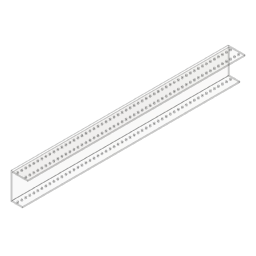
Drivebase Frame v4 (Autodesk Fusion 360 design; units mm, degrees)
Autodesk Fusion 360 part; units mm, degrees
sketch "Sketch1" plane through (0, 0, 0) normal (0, 1, 0) x (1, 0, 0)
  line L0 (-20.3201, -44.3567) -> (29.6862, -44.3567)
  line L1 (13.0174, 33.4308) -> (-20.3201, 33.4308)
  line L2 (-20.3201, 33.4308) -> (-20.3201, -44.3567)
  line L3 (13.0174, 36.6058) -> (-23.4951, 36.6058)
  line L4 (-23.4951, 36.6058) -> (-23.4951, -47.5317)
  line L5 (-23.4951, -47.5317) -> (29.6862, -47.5317)
  line L6 (-23.495, 33.4308) -> (-23.495, 36.6058)
  line L7 (13.0174, 36.6058) -> (13.0174, 33.4308)
  line L8 (29.6862, -47.5317) -> (29.6862, -44.3567)
  dimension "d4" = 53.1812
  dimension "d5" = 84.1375
  dimension "d6" = 36.5125
  constraint horizontal L0
  constraint horizontal L1
  constraint vertical L2
  constraint coincident L1 L6.start
  constraint coincident L3 L6.end
  constraint perpendicular L3 L6
  constraint perpendicular L1 L7
  measures "d4" distance of L4.end L5.end
  measures "d5" distance of L3.end L4.end
  measures "d6" distance of L3.start L3.end
extrude "Extrude1" add sketch "Sketch1" along normal blind 687.3875
sketch "Sketch2" plane through (0, 0, 47.5317) normal (0, 0, 1) x (-1, 0, 0)
  line L0 (23.4951, 0) -> (-29.6862, 0)
  line L1 (-29.6862, 0) -> (-29.6862, -687.3875)
  line L2 (-29.6862, -687.3875) -> (23.4951, -687.3875)
  line L3 (23.4951, -687.3875) -> (23.4951, 0)
  circle A0 centre (-16.9862, -6.35) radius 2.3813
  circle A1 centre (8.4138, -6.35) radius 2.3813
  circle A2 centre (-16.9862, -19.05) radius 2.3813
  circle A3 centre (8.4138, -19.05) radius 2.3813
  circle A4 centre (-16.9862, -31.75) radius 2.3813
  circle A5 centre (8.4138, -31.75) radius 2.3813
  circle A6 centre (-16.9862, -44.45) radius 2.3813
  circle A7 centre (8.4138, -44.45) radius 2.3813
  circle A8 centre (-16.9862, -57.15) radius 2.3813
  circle A9 centre (8.4138, -57.15) radius 2.3813
  circle A10 centre (-16.9862, -69.85) radius 2.3813
  circle A11 centre (8.4138, -69.85) radius 2.3813
  circle A12 centre (-16.9862, -82.55) radius 2.3813
  circle A13 centre (8.4138, -82.55) radius 2.3813
  circle A14 centre (-16.9862, -95.25) radius 2.3813
  circle A15 centre (8.4138, -95.25) radius 2.3813
  circle A16 centre (-16.9862, -107.95) radius 2.3813
  circle A17 centre (8.4138, -107.95) radius 2.3813
  circle A18 centre (-16.9862, -120.65) radius 2.3813
  circle A19 centre (8.4138, -120.65) radius 2.3813
  circle A20 centre (-16.9862, -133.35) radius 2.3813
  circle A21 centre (8.4138, -133.35) radius 2.3813
  circle A22 centre (-16.9862, -146.05) radius 2.3813
  circle A23 centre (8.4138, -146.05) radius 2.3813
  circle A24 centre (-16.9862, -158.75) radius 2.3813
  circle A25 centre (8.4138, -158.75) radius 2.3813
  circle A26 centre (-16.9862, -171.45) radius 2.3813
  circle A27 centre (8.4138, -171.45) radius 2.3813
  circle A28 centre (-16.9862, -184.15) radius 2.3813
  circle A29 centre (8.4138, -184.15) radius 2.3813
  circle A30 centre (-16.9862, -196.85) radius 2.3813
  circle A31 centre (8.4138, -196.85) radius 2.3813
  circle A32 centre (-16.9862, -209.55) radius 2.3813
  circle A33 centre (8.4138, -209.55) radius 2.3813
  circle A34 centre (-16.9862, -222.25) radius 2.3813
  circle A35 centre (8.4138, -222.25) radius 2.3813
  circle A36 centre (-16.9862, -234.95) radius 2.3813
  circle A37 centre (8.4138, -234.95) radius 2.3813
  circle A38 centre (-16.9862, -247.65) radius 2.3813
  circle A39 centre (8.4138, -247.65) radius 2.3813
  circle A40 centre (-16.9862, -260.35) radius 2.3813
  circle A41 centre (8.4138, -260.35) radius 2.3813
  circle A42 centre (-16.9862, -273.05) radius 2.3813
  circle A43 centre (8.4138, -273.05) radius 2.3813
  circle A44 centre (-16.9862, -285.75) radius 2.3813
  circle A45 centre (8.4138, -285.75) radius 2.3813
  circle A46 centre (-16.9862, -298.45) radius 2.3813
  circle A47 centre (8.4138, -298.45) radius 2.3813
  circle A48 centre (-16.9862, -311.15) radius 2.3813
  circle A49 centre (8.4138, -311.15) radius 2.3813
  circle A50 centre (-16.9862, -323.85) radius 2.3813
  circle A51 centre (8.4138, -323.85) radius 2.3813
  circle A52 centre (-16.9862, -336.55) radius 2.3813
  circle A53 centre (8.4138, -336.55) radius 2.3813
  circle A54 centre (-16.9862, -349.25) radius 2.3813
  circle A55 centre (8.4138, -349.25) radius 2.3813
  circle A56 centre (-16.9862, -361.95) radius 2.3813
  circle A57 centre (8.4138, -361.95) radius 2.3813
  circle A58 centre (-16.9862, -374.65) radius 2.3813
  circle A59 centre (8.4138, -374.65) radius 2.3813
  circle A60 centre (-16.9862, -387.35) radius 2.3813
  circle A61 centre (8.4138, -387.35) radius 2.3813
  circle A62 centre (-16.9862, -400.05) radius 2.3813
  circle A63 centre (8.4138, -400.05) radius 2.3813
  circle A64 centre (-16.9862, -412.75) radius 2.3813
  circle A65 centre (8.4138, -412.75) radius 2.3813
  circle A66 centre (-16.9862, -425.45) radius 2.3813
  circle A67 centre (8.4138, -425.45) radius 2.3813
  circle A68 centre (-16.9862, -438.15) radius 2.3813
  circle A69 centre (8.4138, -438.15) radius 2.3813
  circle A70 centre (-16.9862, -450.85) radius 2.3813
  circle A71 centre (8.4138, -450.85) radius 2.3813
  circle A72 centre (-16.9862, -463.55) radius 2.3813
  circle A73 centre (8.4138, -463.55) radius 2.3813
  circle A74 centre (-16.9862, -476.25) radius 2.3813
  circle A75 centre (8.4138, -476.25) radius 2.3813
  circle A76 centre (-16.9862, -488.95) radius 2.3813
  circle A77 centre (8.4138, -488.95) radius 2.3813
  circle A78 centre (-16.9862, -501.65) radius 2.3813
  circle A79 centre (8.4138, -501.65) radius 2.3813
  circle A80 centre (-16.9862, -514.35) radius 2.3813
  circle A81 centre (8.4138, -514.35) radius 2.3813
  circle A82 centre (-16.9862, -527.05) radius 2.3813
  circle A83 centre (8.4138, -527.05) radius 2.3813
  circle A84 centre (-16.9862, -539.75) radius 2.3813
  circle A85 centre (8.4138, -539.75) radius 2.3813
  circle A86 centre (-16.9862, -552.45) radius 2.3813
  circle A87 centre (8.4138, -552.45) radius 2.3813
  circle A88 centre (-16.9862, -565.15) radius 2.3813
  circle A89 centre (8.4138, -565.15) radius 2.3813
  circle A90 centre (-16.9862, -577.85) radius 2.3813
  circle A91 centre (8.4138, -577.85) radius 2.3813
  circle A92 centre (-16.9862, -590.55) radius 2.3813
  circle A93 centre (8.4138, -590.55) radius 2.3813
  circle A94 centre (-16.9862, -603.25) radius 2.3813
  circle A95 centre (8.4138, -603.25) radius 2.3813
  circle A96 centre (-16.9862, -615.95) radius 2.3813
  circle A97 centre (8.4138, -615.95) radius 2.3813
  circle A98 centre (-16.9862, -628.65) radius 2.3813
  circle A99 centre (8.4138, -628.65) radius 2.3813
  circle A100 centre (-16.9862, -641.35) radius 2.3813
  circle A101 centre (8.4138, -641.35) radius 2.3813
  circle A102 centre (-16.9862, -654.05) radius 2.3813
  circle A103 centre (8.4138, -654.05) radius 2.3813
  circle A104 centre (-16.9862, -666.75) radius 2.3813
  circle A105 centre (8.4138, -666.75) radius 2.3813
  circle A106 centre (-16.9862, -679.45) radius 2.3813
  circle A107 centre (8.4138, -679.45) radius 2.3813
  dimension "d9" = 4.7625
  dimension "d12" = 25.4
  dimension "d13" = -12.7
  measures "d9" diameter of A0
hole "Hole1" at (16.9862, 6.35, 47.5317) direction (0, 0, -1) diameter 4.7752 depth 4.7752 tip angle 118
pattern_linear "R-Pattern1" count 54 spacing 12.7 along (0, 1, 0) count 2 spacing 25.4 along (-1, 0, 0) of "Hole1"
sketch "Sketch3" plane through (0, 0, -36.6058) normal (0, 0, -1) x (1, 0, 0)
  line L0 (13.0174, 0) -> (-23.4951, 0)
  line L1 (-23.4951, 0) -> (-23.4951, -687.3875)
  line L2 (-23.4951, -687.3875) -> (13.0174, -687.3875)
  line L3 (13.0174, -687.3875) -> (13.0174, 0)
  circle A0 centre (-8.4075, -6.35) radius 2.3813
  circle A1 centre (-8.4075, -19.05) radius 2.3813
  circle A2 centre (-8.4075, -31.75) radius 2.3813
  circle A3 centre (-8.4075, -44.45) radius 2.3813
  circle A4 centre (-8.4075, -57.15) radius 2.3813
  circle A5 centre (-8.4075, -69.85) radius 2.3813
  circle A6 centre (-8.4075, -82.55) radius 2.3813
  circle A7 centre (-8.4075, -95.25) radius 2.3813
  circle A8 centre (-8.4075, -107.95) radius 2.3813
  circle A9 centre (-8.4075, -120.65) radius 2.3813
  circle A10 centre (-8.4075, -133.35) radius 2.3813
  circle A11 centre (-8.4075, -146.05) radius 2.3813
  circle A12 centre (-8.4075, -158.75) radius 2.3813
  circle A13 centre (-8.4075, -171.45) radius 2.3813
  circle A14 centre (-8.4075, -184.15) radius 2.3813
  circle A15 centre (-8.4075, -196.85) radius 2.3813
  circle A16 centre (-8.4075, -209.55) radius 2.3813
  circle A17 centre (-8.4075, -222.25) radius 2.3813
  circle A18 centre (-8.4075, -234.95) radius 2.3813
  circle A19 centre (-8.4075, -247.65) radius 2.3813
  circle A20 centre (-8.4075, -260.35) radius 2.3813
  circle A21 centre (-8.4075, -273.05) radius 2.3813
  circle A22 centre (-8.4075, -285.75) radius 2.3813
  circle A23 centre (-8.4075, -298.45) radius 2.3813
  circle A24 centre (-8.4075, -311.15) radius 2.3813
  circle A25 centre (-8.4075, -323.85) radius 2.3813
  circle A26 centre (-8.4075, -336.55) radius 2.3813
  circle A27 centre (-8.4075, -349.25) radius 2.3813
  circle A28 centre (-8.4075, -361.95) radius 2.3813
  circle A29 centre (-8.4075, -374.65) radius 2.3813
  circle A30 centre (-8.4075, -387.35) radius 2.3813
  circle A31 centre (-8.4075, -400.05) radius 2.3813
  circle A32 centre (-8.4075, -412.75) radius 2.3813
  circle A33 centre (-8.4075, -425.45) radius 2.3813
  circle A34 centre (-8.4075, -438.15) radius 2.3813
  circle A35 centre (-8.4075, -450.85) radius 2.3813
  circle A36 centre (-8.4075, -463.55) radius 2.3813
  circle A37 centre (-8.4075, -476.25) radius 2.3813
  circle A38 centre (-8.4075, -488.95) radius 2.3813
  circle A39 centre (-8.4075, -501.65) radius 2.3813
  circle A40 centre (-8.4075, -514.35) radius 2.3813
  circle A41 centre (-8.4075, -527.05) radius 2.3813
  circle A42 centre (-8.4075, -539.75) radius 2.3813
  circle A43 centre (-8.4075, -552.45) radius 2.3813
  circle A44 centre (-8.4075, -565.15) radius 2.3813
  circle A45 centre (-8.4075, -577.85) radius 2.3813
  circle A46 centre (-8.4075, -590.55) radius 2.3813
  circle A47 centre (-8.4075, -603.25) radius 2.3813
  circle A48 centre (-8.4075, -615.95) radius 2.3813
  circle A49 centre (-8.4075, -628.65) radius 2.3813
  circle A50 centre (-8.4075, -641.35) radius 2.3813
  circle A51 centre (-8.4075, -654.05) radius 2.3813
  circle A52 centre (-8.4075, -666.75) radius 2.3813
  circle A53 centre (-8.4075, -679.45) radius 2.3813
  dimension "d21" = 4.7625
  dimension "d24" = 0
  dimension "d25" = -12.7
  measures "d21" diameter of A0
hole "Hole2" at (-8.4075, 44.45, -36.6058) at (-8.4075, 400.05, -36.6058) at (-8.4075, 209.55, -36.6058) at (-8.4075, 234.95, -36.6058) at (-8.4075, 463.55, -36.6058) at (-8.4075, 273.05, -36.6058) at (-8.4075, 158.75, -36.6058) at (-8.4075, 184.15, -36.6058) at (-8.4075, 57.15, -36.6058) at (-8.4075, 260.35, -36.6058) at (-8.4075, 6.35, -36.6058) at (-8.4075, 336.55, -36.6058) at (-8.4075, 666.75, -36.6058) at (-8.4075, 196.85, -36.6058) at (-8.4075, 527.05, -36.6058) at (-8.4075, 679.45, -36.6058) at (-8.4075, 565.15, -36.6058) at (-8.4075, 171.45, -36.6058) at (-8.4075, 615.95, -36.6058) at (-8.4075, 361.95, -36.6058) at (-8.4075, 539.75, -36.6058) at (-8.4075, 323.85, -36.6058) at (-8.4075, 552.45, -36.6058) at (-8.4075, 298.45, -36.6058) at (-8.4075, 247.65, -36.6058) at (-8.4075, 107.95, -36.6058) at (-8.4075, 374.65, -36.6058) at (-8.4075, 120.65, -36.6058) at (-8.4075, 412.75, -36.6058) at (-8.4075, 425.45, -36.6058) at (-8.4075, 577.85, -36.6058) at (-8.4075, 69.85, -36.6058) at (-8.4075, 133.35, -36.6058) at (-8.4075, 311.15, -36.6058) at (-8.4075, 501.65, -36.6058) at (-8.4075, 450.85, -36.6058) at (-8.4075, 285.75, -36.6058) at (-8.4075, 146.05, -36.6058) at (-8.4075, 488.95, -36.6058) at (-8.4075, 222.25, -36.6058) at (-8.4075, 654.05, -36.6058) at (-8.4075, 590.55, -36.6058) at (-8.4075, 82.55, -36.6058) at (-8.4075, 603.25, -36.6058) at (-8.4075, 31.75, -36.6058) at (-8.4075, 387.35, -36.6058) at (-8.4075, 19.05, -36.6058) at (-8.4075, 514.35, -36.6058) at (-8.4075, 476.25, -36.6058) at (-8.4075, 349.25, -36.6058) at (-8.4075, 628.65, -36.6058) at (-8.4075, 438.15, -36.6058) at (-8.4075, 641.35, -36.6058) at (-8.4075, 95.25, -36.6058) direction (0, 0, 1) diameter 4.7625 depth 6.35 tip angle 180
component "Drivebase Frame Outside Runner" placed x (1, 0, 0) y (0, 1, 0) z (0, 0, 1) at (0, 0, 0)
equation "d4 = ( 33.5 / 16 ) * 1 in"
equation "d5 = ( 53 / 16 ) * 1 in"
equation "d6 = ( 23 / 16 ) * 1 in"
equation "d9 = ( 3 / 16 ) * 1 in"
equation "d21 = ( 3 / 16 ) * 1 in"
equation "d27 = ( 3 / 16 ) * 1 in"
